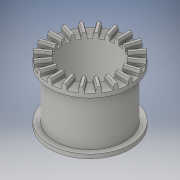
# Autodesk Inventor part: Rigid gears
Saved by Autodesk Inventor 2016 SP1 (Build 200210100, 210)
## iProperties
Created: 2016-02-19
Part Number: Rigid gears
Material: Generic
Document SubType Name: Modeling
Designer: Tore Den Store
Density: 1 g/cm^3
Appearance: Default
Author: Tore Den Store
Autodesk Inventor part; units mm, degrees
ref_plane "YZ Plane" through (0, 0, 0) normal (1, 0, 0) x (0, 1, 0)
sketch "Sketch1" plane through (0, 0, 0) normal (0, 0, 1) x (1, 0, 0)
  circle A0 centre (0, 0) radius 130
  dimension "d0" = 260
  constraints: 1 centre point, 1 coincident
  measures "d0" diameter of A0
extrude "Extrusion1" add sketch "Sketch1" along normal blind 180
sketch "Sketch2" plane through (0, 0, 180) normal (0, 0, 1) x (1, 0, 0)
  circle A0 centre (0, 0) radius 150
  dimension "d3" = 300
  constraints: 1 centre point, 1 coincident
  measures "d3" diameter of A0
extrude "Extrusion2" add sketch "Sketch2" along normal blind 15
ref_plane "Work Plane3" through (0, 0, 90) normal (0, 0, -1) x (-1, 0, 0)
mirror "Mirror2" about plane through (0, 0, 90) normal (0, 0, -1) of "Extrusion2"
hole "Hole2" at (0, 0, 195) direction (0, 0, -1) diameter 200 end through all
sketch "Sketch7" plane through (0, 0, 195) normal (0, 0, 1) x (1, 0, 0)
  circle A0 centre (0, 0) radius 100 projected
  circle A1 centre (0, 0) radius 100 projected
  circle A2 centre (0, 0) radius 150 projected
  line L0 (0, 0) -> (-7.8459, -99.6917) construction
  circle A3 centre (0, 0) radius 150 projected
  line L1 (0, 0) -> (150, 0) construction
  line L2 (0, 0) -> (7.8459, -99.6917) construction
  line L3 (-7.8459, -99.6917) -> (-7.8459, -149.7947)
  line L4 (7.8459, -99.6917) -> (7.8459, -149.7947)
  dimension "d40" = 94.5
  dimension "d41" = 9
  constraints: 10 end point, 6 point on circle, 2 vertical, 1 horizontal
  measures "d40" angle of L0 L1
  measures "d41" angle of L2 L0
extrude "Extrusion7" add sketch "Sketch7" along normal blind 20 contours A0 L4 A2 L3 picked at (6.1032, -116.484)
ref_plane "Work Plane4" through (-7.8459, -149.7947, 195) normal (0, 1, 0) x (0, 0, 1)
sketch "Sketch8" plane through (-7.8459, -149.7947, 195) normal (0, 1, 0) x (0, 0, 1)
  line L0 (20, 15.6918) -> (20, 0) projected
  line L1 (20, 0) -> (10, 0)
  line L2 (0, 0) -> (20, 0) projected
  line L3 (20, 0) -> (20, 3.6397)
  line L4 (10, 0) -> (20, 3.6397)
  line L5 (0, 15.6918) -> (20, 15.6918) projected
  line L6 (20, 15.6918) -> (10, 15.6918)
  line L7 (10, 15.6918) -> (20, 12.0521)
  line L8 (20, 12.0521) -> (20, 15.6918)
  point P0 (-195, 7.8459)
  dimension "d49" = 10
  dimension "d50" = 20
  dimension "d52" = 10
  dimension "d53" = 20
  constraints: 12 end point, 2 midpoint, 2 point on line, 1 collinear
  measures "d49" distance of L0.end L1.end
  measures "d50" angle of L4 L1
  measures "d52" distance of L0.start L6.end
  measures "d53" angle of L5 L7
extrude "Extrusion8" cut sketch "Sketch8" along normal through all both and the other way through all
pattern_circular "Circular Pattern1" count 20 over 360 about axis through (0, 0, -278.392) along (0, 0, 1) of "Extrusion8", "Extrusion7"
equation "\"d52\" = d49"
equation "\"d53\" = d50"
body "Solid1"
